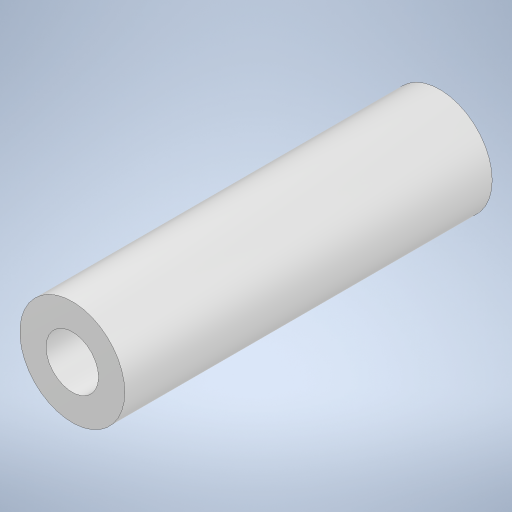
# Autodesk Inventor part: PEAKスペーサーm3中空-17
Saved by Autodesk Inventor 2023 (Build 270158030, 158C)
## iProperties
Created: 2020-05-12
Part Number: PEAKスペーサーm3中空-17
Material: アルミニウム 2014-T6
Document SubType Name: Modeling
Designer: mozar
Density: 2.78927 g/cm^3
Appearance: サテン
Mass: 0.475857 g
Surface Area: 5.23075 cm^2
Volume: 0.360498 cm^3
Author: mozar
Autodesk Inventor part; units mm, degrees
ref_plane "YZ Plane" through (0, 0, 0) normal (1, 0, 0) x (0, 1, 0)
ref_plane "XZ Plane" through (0, 0, 0) normal (0, 1, 0) x (-1, 0, 0)
ref_plane "XY Plane" through (0, 0, 0) normal (0, 0, 1) x (1, 0, 0)
sketch "スケッチ1" plane through (0, 0, 0) normal (0, 0, 1) x (1, 0, 0)
  circle A0 centre (0, 0) radius 3
  circle A1 centre (0, 0) radius 1.5
  dimension "d0" = 6
  dimension "d1" = 3
  constraints: 2 centre point, 2 coincident
  measures "d0" diameter of A0
  measures "d1" diameter of A1
extrude "押し出し1" add sketch "スケッチ1" against normal blind 21
